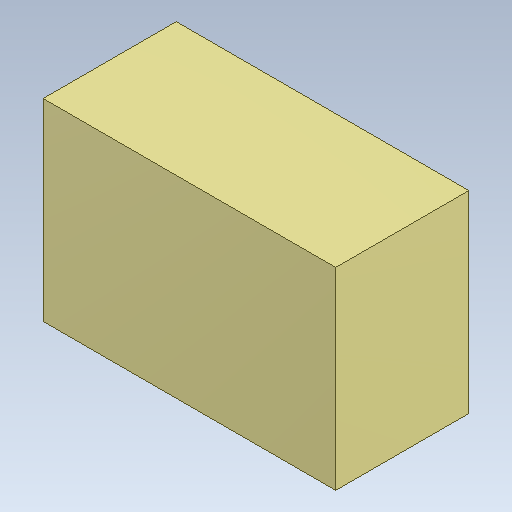
# Autodesk Inventor part: 10UF
Saved by Autodesk Inventor 2020 (Build 240168000, 168)
## iProperties
Created: 2019-05-24
Part Number: 10UF
Material: Generic
Document SubType Name: Modeling
Designer: psrob
Density: 1 g/cm^3
Appearance: 0805-NO, 10UF
Author: psrob
Autodesk Inventor part; units mm, degrees
ref_plane "YZ Plane" through (0, 0, 0) normal (1, 0, 0) x (0, 1, 0)
ref_plane "XZ Plane" through (0, 0, 0) normal (0, 1, 0) x (-1, 0, 0)
ref_plane "XY Plane" through (0, 0, 0) normal (0, 0, 1) x (1, 0, 0)
sketch "0805-NO, 10UF_9" plane through (0, 0, 0) normal (0, 0, 1) x (1, 0, 0)
  line L0 (-1.0922, 0.7262) -> (1.1057, 0.7262)
  line L1 (1.1057, 0.7262) -> (1.1057, -0.7239)
  line L2 (1.1057, -0.7239) -> (-1.0922, -0.7239)
  line L3 (-1.0922, -0.7239) -> (-1.0922, 0.7262)
  constraints: 8 end point
extrude "Extrusion1" add sketch "0805-NO, 10UF_9" along normal blind 1
body "Solid1"
